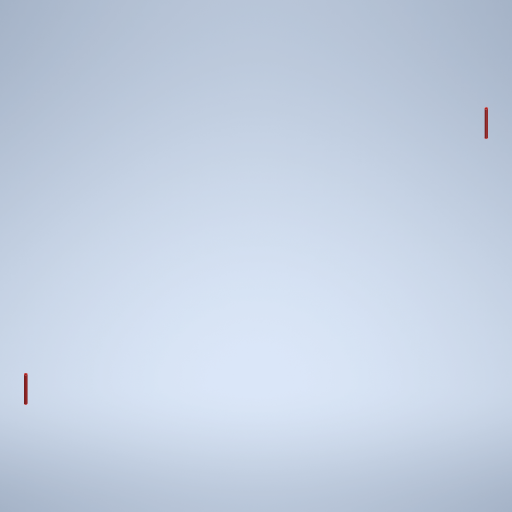
# Autodesk Inventor part: Rafix Skeleton
Saved by Autodesk Inventor 2024 (Build 280153000, 153)
## iProperties
RuleStatus: InUse
Created: 2023-03-16
Part Number: Rafix Skeleton
Material: Generic
Document SubType Name: Modeling
Designer: sauliusd
Density: 1 g/cm^3
Appearance: Default
AfterAnyParamChange0: Parameters Control
AfterAnyUserParamChange0: Parameters Control
Author: sauliusd
Autodesk Inventor part; units mm, degrees
ref_plane "YZ Plane" through (0, 0, 0) normal (1, 0, 0) x (0, 1, 0)
ref_plane "XZ Plane" through (0, 0, 0) normal (0, 1, 0) x (-1, 0, 0)
ref_plane "XY Plane" through (0, 0, 0) normal (0, 0, 1) x (1, 0, 0)
sketch "Sketch1" plane through (0, 0, 0) normal (0, 0, 1) x (1, 0, 0)
  line L0 (-150, -8) -> (150, -8)
  line L1 (150, -8) -> (150, 8)
  line L2 (150, 8) -> (-150, 8)
  line L3 (-150, 8) -> (-150, -8)
  line L4 (-150, -8) -> (150, 8) construction
  line L5 (150, -8) -> (-150, 8) construction
  circle A0 centre (-90, 0) radius 0.5
  point P0 (0, 0)
  point P1 (90, 0)
  dimension "ContactPatchLength" = 300
  dimension "ContactPatchWidth" = 16
  dimension "Offset1" = 60
  dimension "Offset2" = 60
  dimension "YCoord" = 8
  dimension "d5" = 1
  constraints: 12 end point, 2 midpoint, 2 parallel, 1 centre point, 1 coincident, 1 horizontal, 1 horizontal alignment, 1 perpendicular
  measures "ContactPatchLength" distance of L2.end L1.end
  measures "ContactPatchWidth" distance of L1.end L0.end
  measures "Offset1" distance from line of point (-90, 0) L3
  measures "Offset2" distance from line of L1 point (90, 0)
  measures "YCoord" distance from line of L2 point (-90, 0)
  measures "d5" diameter of A0
extrude "Extrusion1" add sketch "Sketch1" along normal blind 10 contours A0
pattern_linear "Rectangular Pattern1" count 2 spacing 180 along (1, 0, 0) of "Extrusion1"
equation "\"d10\" = SpaceBetween"
equation "\"SpaceBetween\" = 180"
equation "\"MinDistance\" = 32"
body "Solid1"
